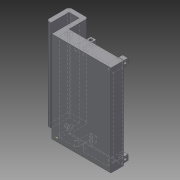
# Autodesk Inventor part: base
Saved by Autodesk Inventor 2015 (Build 190159000, 159)
## iProperties
Created: 2019-01-19
Part Number: base
Material: Generic
Document SubType Name: Modeling
Designer: Toby
Density: 1 g/cm^3
Appearance: Default
Author: Toby
Autodesk Inventor part; units mm, degrees
ref_plane "YZ Plane" through (0, 0, 0) normal (1, 0, 0) x (0, 1, 0)
ref_plane "XZ Plane" through (0, 0, 0) normal (0, 1, 0) x (-1, 0, 0)
ref_plane "XY Plane" through (0, 0, 0) normal (0, 0, 1) x (1, 0, 0)
sketch "Sketch1" plane through (0, 0, 0) normal (0, 0, 1) x (1, 0, 0)
  line L0 (-17.8652, 22.0745) -> (-12.8652, 22.0745)
  line L1 (-12.8652, 22.0745) -> (-12.8652, -2.9255)
  line L2 (-12.8652, -2.9255) -> (-17.8652, -2.9255)
  line L3 (-17.8652, -2.9255) -> (-17.8652, 22.0745)
  line L4 (-12.8652, 22.0745) -> (3.1348, 22.0745)
  line L5 (3.1348, 22.0745) -> (3.1348, 17.0745)
  line L6 (3.1348, 17.0745) -> (-12.8652, 17.0745)
  line L7 (-12.8652, 17.0745) -> (-12.8652, 22.0745)
  line L8 (3.1348, 17.0745) -> (-1.8652, 17.0745)
  line L9 (-1.8652, 17.0745) -> (-1.8652, -12.9255)
  line L10 (-1.8652, -12.9255) -> (3.1348, -12.9255)
  line L11 (3.1348, -12.9255) -> (3.1348, 17.0745)
  line L12 (3.1348, -12.9255) -> (63.1348, -12.9255)
  line L13 (63.1348, -12.9255) -> (63.1348, -8.9255)
  line L14 (63.1348, -8.9255) -> (3.1348, -8.9255)
  line L15 (3.1348, -8.9255) -> (3.1348, -12.9255)
  point P0 (0, 0)
  dimension "d0" = 11
  dimension "d1" = 5
  dimension "d2" = 5
  dimension "d3" = 20
  dimension "d4" = 30
  dimension "d5" = 5
  dimension "d6" = 4
  dimension "d7" = 60
  constraints: 32 end point, 8 parallel, 4 horizontal, 4 perpendicular
  measures "d0" distance between parallel lines of L9 L1
  measures "d1" distance between parallel lines of L4 L6
  measures "d2" distance between parallel lines of L3 L1
  measures "d3" distance between parallel lines of L2 L6
  measures "d4" distance between parallel lines of L10 L8
  measures "d5" distance between parallel lines of L11 L9
  measures "d6" distance between parallel lines of L12 L14
  measures "d7" distance between parallel lines of L15 L13
extrude "Extrusion1" add sketch "Sketch1" along normal blind 100
sketch "Sketch2" plane through (3.1348, -8.9255, 0) normal (1, 0, 0) x (0, 0, -1)
  line L0 (0, 26) -> (-100, 26) projected
  point P0 (0, 8.9255)
  point P1 (-92.9382, 11)
  point P2 (-5.6681, 11)
  dimension "d10" = 15
  dimension "d11" = 15
  measures "d10" distance from line of L0 point (-92.938, 11)
  measures "d11" distance from line of L0 point (-5.668, 11)
hole "Hole1" at (3.1348, 2.0745, 92.9382) at (3.1348, 2.0745, 5.6681) direction (-1, 0, 0) diameter 3 depth 8 tip angle 118 countersink diameter 6 countersink angle 90
chamfer "Chamfer1" distance 2 angle 45 2 edges at (-17.8652, 22.0745, 50) (-17.8652, -2.9255, 50)
chamfer "Chamfer2" distance 2 angle 45 1 edges at (3.1348, 22.0745, 50)
sketch "Sketch3" plane through (3.1348, -8.9255, 0) normal (0, 1, 0) x (1, 0, 0)
  point P0 (-3.1348, 0)
sketch "Sketch4" plane through (3.1348, -8.9255, 0) normal (0, 1, 0) x (1, 0, 0)
  line L0 (0, -100) -> (60, -100)
  line L1 (60, -100) -> (60, -98.8)
  line L2 (60, -98.8) -> (0, -98.8)
  line L3 (0, -98.8) -> (0, -100)
  line L4 (-5, 0) -> (60, 0) projected
  line L5 (60, -98.8) -> (58.8, -98.8)
  line L6 (58.8, -98.8) -> (58.8, 0)
  line L7 (58.8, 0) -> (60, 0)
  line L8 (60, 0) -> (60, -98.8)
  line L9 (0, 0) -> (58.8, 0)
  line L10 (58.8, 0) -> (58.8, -1.2)
  line L11 (58.8, -1.2) -> (0, -1.2)
  line L12 (0, -1.2) -> (0, 0)
  line L13 (60, 0) -> (60, -100) projected
  point P0 (-3.1348, 0)
  dimension "d25" = 1.2
  dimension "d26" = 1.2
  dimension "d27" = 1.2
  constraints: 24 end point, 6 parallel, 4 point on line, 3 horizontal, 3 perpendicular, 1 collinear
  measures "d25" distance between parallel lines of L0 L2
  measures "d26" distance between parallel lines of L8 L6
  measures "d27" distance between parallel lines of L4 L11
extrude "Extrusion2" add sketch "Sketch4" along normal blind 10
sketch "Sketch5" plane through (3.1348, -8.9255, 98.8) normal (0, 1, 0) x (1, 0, 0)
  line L0 (58.8, 0) -> (52.8, 0)
  line L1 (52.8, 0) -> (52.8, 6)
  line L2 (52.8, 6) -> (58.8, 6)
  line L3 (58.8, 6) -> (58.8, 0)
  line L4 (58.8, 97.6) -> (52.8, 97.6)
  line L5 (52.8, 97.6) -> (52.8, 91.6)
  line L6 (52.8, 91.6) -> (58.8, 91.6)
  line L7 (58.8, 91.6) -> (58.8, 97.6)
  point P0 (-3.1348, 98.8)
  dimension "d30" = 6
  dimension "d31" = 6
  dimension "d32" = 6
  dimension "d33" = 6
  constraints: 16 end point, 4 parallel, 2 horizontal, 2 perpendicular
  measures "d30" distance of L1.end L2.end
  measures "d31" distance of L0.end L1.end
  measures "d32" distance of L6.end L5.end
  measures "d33" distance of L5.end L4.end
extrude "Extrusion3" add sketch "Sketch5" along normal blind 16
sketch "Sketch6" plane through (61.9348, 1.0745, 1.2) normal (1, 0, 0) x (0, 0, -1)
  line L0 (-6, 6) -> (0, 6) projected
  line L1 (0, 0) -> (0, 6) projected
  line L2 (-97.6, 6) -> (-91.6, 6) projected
  line L3 (-97.6, 0) -> (-97.6, 6) projected
  point P0 (1.2, -1.0745)
  point P1 (-94.6, 3)
  point P2 (-3, 3)
  dimension "d36" = 3
  dimension "d37" = 3
  dimension "d38" = 3
  dimension "d39" = 3
  measures "d36" distance from line of L0 point (-3, 3)
  measures "d37" distance from line of L1 point (-3, 3)
  measures "d38" distance from line of L2 point (-94.6, 3)
  measures "d39" distance from line of L3 point (-94.6, 3)
hole "Hole2" at (61.9348, 4.0745, 95.8) at (61.9348, 4.0745, 4.2) direction (-1, 0, 0) diameter 3 depth 8 tip angle 118
sketch "Sketch7" plane through (3.1348, -8.9255, 98.8) normal (0, 1, 0) x (1, 0, 0)
  line L0 (0, 0) -> (52.8, 0) projected
  line L1 (18, 0) -> (24, 0)
  line L2 (24, 0) -> (24, 6)
  line L3 (24, 6) -> (18, 6)
  line L4 (18, 6) -> (18, 0)
  line L5 (52.8, 97.6) -> (0, 97.6) projected
  line L6 (18, 97.6) -> (24, 97.6)
  line L7 (24, 97.6) -> (24, 91.6)
  line L8 (24, 91.6) -> (18, 91.6)
  line L9 (18, 91.6) -> (18, 97.6)
  line L10 (0, -1.2) -> (0, 98.8) projected
  point P0 (-3.1348, 98.8)
  dimension "d47" = 6
  dimension "d48" = 6
  dimension "d49" = 6
  dimension "d50" = 6
  dimension "d51" = 18
  constraints: 16 end point, 4 parallel, 3 point on line, 2 horizontal, 2 perpendicular
  measures "d47" distance of L3.end L2.end
  measures "d48" distance of L2.end L1.end
  measures "d49" distance of L7.end L8.end
  measures "d50" distance of L6.end L7.end
  measures "d51" distance between parallel lines of L10 L4
extrude "Extrusion4" add sketch "Sketch7" along normal blind 16
sketch "Sketch8" plane through (21.1348, 1.0745, 98.8) normal (0, 0, 1) x (1, 0, 0)
  line L0 (6, 6) -> (0, 6) projected
  point P0 (-21.1348, -1.0745)
  point P1 (3, 3)
  dimension "d54" = 3
  measures "d54" distance from line of L0 point (3, 3)
hole "Hole3" at (24.1348, 4.0745, 98.8) direction (0, 0, -1) diameter 3 depth 800 tip angle 118
chamfer "Chamfer3" distance 2 angle 45 4 edges at (27.1348, -8.9255, 4.2) (27.1348, -8.9255, 95.8) (21.1348, -8.9255, 95.8) (21.1348, -8.9255, 4.2)
body "Solid1"
